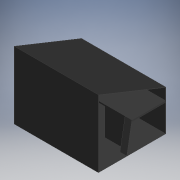
# Autodesk Inventor part: out
Saved by Autodesk Inventor 2017 (Build 210142000, 142)
## iProperties
Created: 2019-10-04
Part Number: out
Material: Generic
Document SubType Name: Modeling
Designer: Ellie
Density: 1 g/cm^3
Appearance: Default
Author: Ellie
Autodesk Inventor part; units mm, degrees
ref_plane "YZ Plane" through (0, 0, 0) normal (1, 0, 0) x (0, 1, 0)
ref_plane "XZ Plane" through (0, 0, 0) normal (0, 1, 0) x (-1, 0, 0)
sketch "Sketch1" plane through (0, 0, 0) normal (0, 1, 0) x (-1, 0, 0)
  line L0 (-3048, 3810) -> (3048, 3810)
  line L1 (3048, 3810) -> (3048, -3810)
  line L2 (3048, -3810) -> (-3048, -3810)
  line L3 (-3048, -3810) -> (-3048, 3810)
  line L4 (-3048, 3810) -> (3048, -3810) construction
  line L5 (3048, 3810) -> (-3048, -3810) construction
  point P0 (0, 0)
  dimension "d0" = 7620
  dimension "d1" = 6096
  constraints: 12 end point, 2 midpoint, 2 parallel, 1 horizontal, 1 perpendicular
  measures "d0" distance of L0.end L1.end
  measures "d1" distance of L1.end L2.end
extrude "main body" add sketch "Sketch1" along normal blind 3657.6
sketch "Sketch3" plane through (0, 0, 0) normal (0, 0, 1) x (1, 0, 0)
  line L0 (-3048, 3657.6) -> (-3048, 6096)
  line L1 (-3048, 6096) -> (3048, 3657.6)
  line L2 (3048, 3657.6) -> (-3048, 3657.6)
  point P0 (0, 0)
  dimension "d4" = 2438.4
  constraints: 6 end point, 2 coincident, 1 vertical
  measures "d4" distance of L0.start L0.end
extrude "triangle" add sketch "Sketch3" along normal mid plane 7620
shell "Shell1" thickness 25.4 removed faces 1 at (-1016, 3251.2, 3810)
ref_plane "Work Plane1" through (-3022.6, 2463.8, 3810) normal (0, 1, 0) x (1, 0, 0)
sketch "Sketch6" plane through (-3022.6, 2463.8, 3810) normal (0, 1, 0) x (1, 0, 0)
  line L0 (6045.2, 0) -> (2997.2, 0)
  line L1 (2997.2, 0) -> (2997.2, 7594.6)
  line L2 (2997.2, 7594.6) -> (6045.2, 7594.6)
  line L3 (6045.2, 7594.6) -> (6045.2, 0)
  point P0 (3022.6, 3810)
  dimension "d12" = 3048
  constraints: 8 end point, 2 parallel, 1 coincident, 1 horizontal, 1 perpendicular
  measures "d12" distance of L0.start L0.end
extrude "second floor" add sketch "Sketch6" along normal blind 152.4
ref_plane "Work Plane3" through (-3022.6, 3073.4, 3810) normal (0, 1, 0) x (1, 0, 0)
sketch "Sketch8" plane through (-3022.6, 3073.4, 3810) normal (0, 1, 0) x (1, 0, 0)
  line L0 (0, 7594.6) -> (2997.2, 7594.6)
  line L1 (2997.2, 7594.6) -> (2997.2, 5461)
  line L2 (2997.2, 5461) -> (0, 5461)
  line L3 (0, 5461) -> (0, 7594.6)
  line L4 (2997.2, 7594.6) -> (2997.2, 0) projected
  line L5 (0, 0) -> (0, 7594.6) projected
  line L6 (2997.2, 7594.6) -> (3606.8, 7594.6)
  line L7 (3606.8, 7594.6) -> (3606.8, 6680.2)
  line L8 (3606.8, 6680.2) -> (2997.2, 6680.2)
  line L9 (2997.2, 6680.2) -> (2997.2, 7594.6)
  point P0 (3022.6, 3810)
  dimension "d17" = 0
  dimension "d19" = 0
  dimension "d20" = 2133.6
  dimension "d23" = 0
  dimension "d39" = 609.6
  dimension "d40" = 914.4
  constraints: 16 end point, 4 parallel, 2 horizontal, 2 perpendicular, 1 collinear
  measures "d17" distance between parallel lines of L4 L1
  measures "d19" distance from line of L0 L5.end
  measures "d20" distance of L0.end L1.end
  measures "d23" distance between parallel lines of L5 L3
  measures "d39" distance of L7.end L8.end
  measures "d40" distance of L6.end L7.end
extrude "bedroom" add sketch "Sketch8" along normal blind 152.4
sketch "Sketch16" plane through (-25.4, 3073.4, -1651) normal (1, 0, 0) x (0, 0, -1)
  line L0 (1219.2, 0) -> (304.8, -457.2)
  line L1 (1219.2, 0) -> (1219.2, 152.4) projected
  line L2 (2133.6, -457.2) -> (-5461, -457.2) projected
  line L3 (0, 0) -> (0, 152.4) projected
  line L4 (1219.2, 152.4) -> (0, -457.2)
  line L5 (2133.6, -457.2) -> (-5461, -457.2) projected
  line L6 (304.8, -457.2) -> (0, -457.2)
  line L7 (1219.2, 152.4) -> (1219.2, 0)
  point P0 (-1651, -3073.4)
  point P1 (-1803.4, -558.8)
  point P2 (-5461, -457.2)
  dimension "d42" = 0
  constraints: 8 end point, 1 horizontal, 1 parallel, 1 vertical, 4 other
  measures "d42" distance from line of L3 L4.end
extrude "upper stairs" add sketch "Sketch16" along normal blind 609.6
sketch "Sketch17" plane through (-3048, 0, 3810) normal (0, 0, 1) x (1, 0, 0)
  line L0 (3022.6, 2463.8) -> (2592.6443, 25.4)
  line L1 (6070.6, 25.4) -> (25.4, 25.4) projected
  line L2 (3022.6, 2616.2) -> (2565.7721, 25.4)
  line L3 (6070.6, 2463.8) -> (3022.6, 2463.8) projected
  line L4 (3022.6, 2463.8) -> (3022.6, 25.4) projected
  line L5 (3022.6, 2616.2) -> (3022.6, 2463.8)
  line L6 (2565.7721, 25.4) -> (2592.6443, 25.4)
  line L7 (3022.6, 2616.2) -> (6070.6, 2616.2) projected
  line L8 (3022.6, 2463.8) -> (3022.6, 2616.2) projected
  line L9 (3022.6, 2616.2) -> (3022.6, 2463.8)
  point P0 (3048, 0)
  dimension "d46" = 100
  constraints: 10 end point, 2 point on line, 1 coincident, 1 collinear, 1 horizontal, 1 parallel, 1 vertical
  measures "d46" angle of L3 L0
extrude "main stairs" add sketch "Sketch17" against normal blind 609.6 contours L0 L1 L2 L5
sketch "Sketch18" plane through (3022.6, 25.4, -3784.6) normal (-1, 0, 0) x (0, 0, 1)
  point P0 (3784.6, -25.4)
ref_plane "Work Plane4" through (0, 0, 1371.6) normal (0, 0, 1) x (1, 0, 0)
sketch "Sketch20" plane through (0, 0, 1371.6) normal (0, 0, 1) x (1, 0, 0)
  line L0 (3022.6, 2463.8) -> (-25.4, 2463.8) projected
  line L1 (3022.6, 25.4) -> (3022.6, 2463.8) projected
  line L2 (-25.4, 2463.8) -> (3022.6, 2463.8)
  line L3 (3022.6, 2463.8) -> (3022.6, 25.4)
  line L4 (3022.6, 25.4) -> (-25.4, 25.4)
  line L5 (-25.4, 25.4) -> (-25.4, 2463.8)
  point P0 (0, 0)
  constraints: 8 end point, 2 parallel, 1 horizontal, 1 perpendicular
extrude "room wall 1" add sketch "Sketch20" along normal blind 50.8
sketch "Sketch21" plane through (-25.4, 2616.2, -3784.6) normal (-1, 0, 0) x (0, 0, 1)
  line L0 (7594.6, -152.4) -> (5207, -152.4) projected
  line L1 (5207, -2590.8) -> (7594.6, -2590.8) projected
  line L2 (5207, -152.4) -> (6985, -152.4)
  line L3 (6985, -152.4) -> (6985, -2590.8)
  line L4 (6985, -2590.8) -> (5207, -2590.8)
  line L5 (5207, -2590.8) -> (5207, -152.4)
  line L6 (6985, -2590.8) -> (6985, 0) projected
  point P0 (3784.6, -2616.2)
  dimension "d55" = 0
  constraints: 8 end point, 2 parallel, 1 horizontal, 1 perpendicular, 1 point on line
  measures "d55" distance between parallel lines of L6 L3
extrude "room wall 2" add sketch "Sketch21" against normal blind 50.8
sketch "Sketch22" plane through (-25.4, 25.4, 3200.4) normal (0, 0, 1) x (1, 0, 0)
  line L0 (3048, 2438.4) -> (0, 2438.4) projected
  line L1 (-429.9557, 0) -> (0, 2438.4) projected
  line L2 (0, 2438.4) -> (-429.9557, 0)
  line L3 (-429.9557, 0) -> (50.8, 0)
  line L4 (50.8, 2438.4) -> (50.8, 0) projected
  line L5 (50.8, 2438.4) -> (50.8, 0)
  line L6 (0, 0) -> (3048, 0) projected
  line L7 (0, 2438.4) -> (50.8, 2438.4)
  point P0 (25.4, -25.4)
  constraints: 8 end point, 2 collinear, 1 horizontal, 1 perpendicular, 1 point on line
extrude "room closet wall" add sketch "Sketch22" along normal blind 50.8
sketch "Sketch23" plane through (-3048, 0, 3810) normal (0, 0, 1) x (1, 0, 0)
  line L0 (0, 0) -> (0, 6096) projected
  line L1 (6096, 0) -> (6096, 3657.6) projected
  line L2 (0, 6096) -> (6096, 3657.6)
  line L3 (6096, 3657.6) -> (6096, 0)
  line L4 (6096, 0) -> (0, 0) projected
  line L5 (6096, 0) -> (0, 0)
  line L6 (6096, 3657.6) -> (0, 6096) projected
  line L7 (0, 0) -> (0, 6096)
  line L8 (2565.7721, 25.4) -> (25.4, 25.4) projected
  point P0 (3048, 0)
  point P1 (25.4, 6058.4834)
  point P2 (6070.6, 3640.4034)
  point P3 (6070.6, 25.4)
  constraints: 8 end point, 2 perpendicular, 1 collinear
extrude "outer wall" [suppressed]
body "Solid1"
